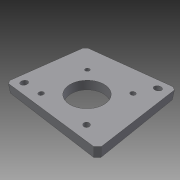
# Autodesk Inventor part: z_rod_stopper_bottom
Saved by Autodesk Inventor 2014 (Build 180170000, 170)
## iProperties
Created: 2013-12-06
Part Number: z_rod_stopper_bottom
Material: Generic
Document SubType Name: Modeling
Designer: buben
Density: 1 g/cm^3
Appearance: Default
Author: buben
Autodesk Inventor part; units mm, degrees
ref_plane "YZ Plane" through (0, 0, 0) normal (1, 0, 0) x (0, 1, 0)
ref_plane "XZ Plane" through (0, 0, 0) normal (0, 1, 0) x (-1, 0, 0)
ref_plane "XY Plane" through (0, 0, 0) normal (0, 0, 1) x (1, 0, 0)
sketch "Sketch1" plane through (0, 0, 0) normal (0, 0, 1) x (1, 0, 0)
  line L0 (20.5, 37.5) -> (51.5, 37.5) construction
  line L1 (51.5, 37.5) -> (51.5, 6.5) construction
  line L2 (51.5, 6.5) -> (20.5, 6.5) construction
  line L3 (20.5, 6.5) -> (20.5, 37.5) construction
  line L4 (14.62, 43.38) -> (57.38, 43.38) construction
  line L5 (57.38, 43.38) -> (57.38, 0.62) construction
  line L6 (57.38, 0.62) -> (14.62, 0.62) construction
  line L7 (14.62, 0.62) -> (14.62, 43.38) construction
  circle A0 centre (20.5, 6.5) radius 1.6
  circle A1 centre (51.5, 6.5) radius 1.6
  circle A2 centre (51.5, 37.5) radius 1.6
  circle A3 centre (20.5, 37.5) radius 1.6
  circle A4 centre (36, 22) radius 11.5
  circle A5 centre (13, 22) radius 4 construction
  circle A6 centre (7, 6) radius 2.25
  circle A7 centre (57.5, 49.5) radius 2.25
  line L8 (2, 56) -> (62, 56)
  line L9 (64, 54) -> (64, 2)
  line L10 (62, 0) -> (2, 0)
  line L11 (0, 2) -> (0, 54)
  line L12 (0, 2) -> (2, 0)
  line L13 (0, 54) -> (2, 56)
  line L14 (62, 56) -> (64, 54)
  line L15 (64, 2) -> (62, 0)
  circle A8 centre (7, 6) radius 4.5 construction
  circle A9 centre (57.5, 49.5) radius 4.5 construction
  point P0 (0, 0)
  point P1 (36, 37.5)
  point P2 (51.5, 22)
  point P3 (14.62, 22)
  point P4 (36, 43.38)
  point P5 (0, 56)
  point P6 (64, 0)
  point P7 (64, 56)
  point P8 (0, 0)
  dimension "d0" = 31
  dimension "d1" = 42.76
  dimension "d2" = 3.2
  dimension "d3" = 23
  dimension "d4" = 8
  dimension "d5" = 23
  dimension "d6" = 4.5
  dimension "d7" = 2
  dimension "d8" = 2
  dimension "d9" = 2
  dimension "d10" = 2
  dimension "d11" = 2
  dimension "d12" = 2
  dimension "d13" = 2
  dimension "d14" = 2
  dimension "d15" = 22
  dimension "d16" = 9
  dimension "d17" = 6
  dimension "d18" = 6
  dimension "d19" = 6
  dimension "d20" = 12
  dimension "d21" = 28
  dimension "d22" = 36
  dimension "d23" = 34
  constraints: 32 end point, 10 centre point, 8 point on line, 7 coincident, 6 parallel, 5 equal radius, 5 perpendicular, 4 midpoint, 3 horizontal, 3 horizontal alignment, 2 vertical alignment
  measures "d0" distance of L1.end L2.end
  measures "d1" distance of L5.end L6.end
  measures "d2" diameter of A0
  measures "d3" diameter of A4
  measures "d4" diameter of A5
  measures "d5" distance of A4.centre A5.centre
  measures "d6" diameter of A6
  measures "d7" distance of L11.start point (0, 0)
  measures "d8" distance of L10.end point (0, 0)
  measures "d9" distance of L11.end point (0, 56)
  measures "d10" distance of L8.start point (0, 56)
  measures "d11" distance of L8.end point (64, 56)
  measures "d12" distance of L9.start point (64, 56)
  measures "d13" distance of L9.end point (64, 0)
  measures "d14" distance of L10.start point (64, 0)
  measures "d15" distance from line of L10 A4.centre
  measures "d16" diameter of A8
  measures "d17" distance from line of L10 A6.centre
  measures "d18" horizontal distance of A5.centre A8.centre
  measures "d19" horizontal distance of L0.end A7.centre
  measures "d20" vertical distance of L0.end A7.centre
  measures "d21" distance from line of L9 A4.centre
  measures "d22" distance from line of L11 A4.centre
  measures "d23" distance from line of L8 A4.centre
extrude "Extrusion1" add sketch "Sketch1" along normal blind 6
equation "\"d8\" = d7"
equation "\"d9\" = d7"
equation "\"d10\" = d9"
equation "\"d11\" = d7"
equation "\"d12\" = d11"
equation "\"d13\" = d7"
equation "\"d14\" = d13"
body "Solid1"
